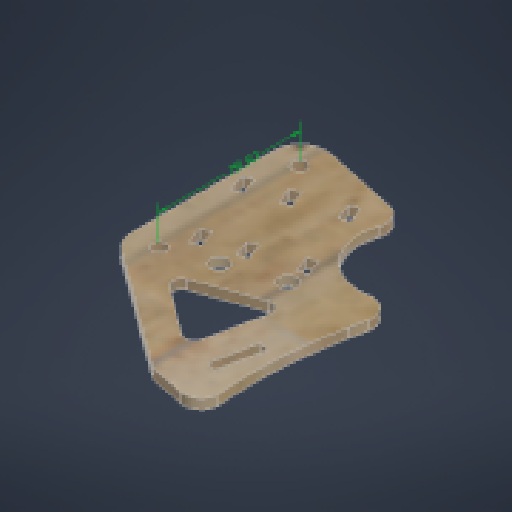
# Autodesk Inventor part: gear_plate_cover
Saved by Autodesk Inventor 2026.3 (Build 303398000, 398)
## iProperties
Created: 2024-04-01
Part Number: gear_plate_cover
Material: 木材 (カエデ材)
Document SubType Name: Modeling
Designer: hibik
Density: 0.67 g/cm^3
Appearance: ナチュラル カエデ材 - 光沢 濃い着色
Author: hibik
Autodesk Inventor part; units mm, degrees
ref_plane "YZ Plane" through (0, 0, 0) normal (1, 0, 0) x (0, 1, 0)
ref_plane "XZ Plane" through (0, 0, 0) normal (0, 1, 0) x (-1, 0, 0)
ref_plane "XY Plane" through (0, 0, 0) normal (0, 0, 1) x (1, 0, 0)
sketch "スケッチ1" plane through (0, 0, 0) normal (0, 1, 0) x (-1, 0, 0)
  line L0 (25, 0) -> (-25, 0)
  line L1 (-25, 0) -> (-25, -104.5)
  line L2 (-25, -104.5) -> (25, -104.5) construction
  line L3 (25, -104.5) -> (25, 0)
  circle A0 centre (0, 0) radius 25
  circle A1 centre (0, 0) radius 57 construction
  circle A2 centre (0, -79.5) radius 22.5 construction
  circle A3 centre (0, 0) radius 75 construction
  circle A4 centre (0, -79.5) radius 4
  circle A5 centre (0, 0) radius 4
  circle A6 centre (-77.7461, -62.8931) radius 25
  circle A7 centre (-77.7461, -62.8931) radius 10.75
  circle A8 centre (0, -79.5) radius 25
  line L4 (-5.2223, -103.9485) -> (-82.9684, -87.3415)
  line L5 (-72.5238, -38.4446) -> (5.2223, -55.0515)
  line L6 (-77.7461, -62.8931) -> (-82.9684, -87.3415)
  point P0 (25, -79.5)
  point P1 (-25, -48.5959)
  dimension "d0" = 114
  dimension "d1" = 45
  dimension "d2" = 150
  dimension "d4" = 8
  dimension "d5" = 50
  dimension "d25" = 79.5
  dimension "d41" = 8
  constraints: 14 end point, 9 centre point, 9 tangent, 8 coincident, 5 point on circle, 2 parallel, 2 perpendicular, 1 equal radius, 1 horizontal, 1 midpoint, 1 vertical alignment
  measures "d0" diameter of A1
  measures "d1" diameter of A2
  measures "d2" diameter of A3
  measures "d4" diameter of A5
  measures "d5" distance of L1.end L2.end
  measures "d25" distance from line of A2.centre L6
  measures "d41" diameter of A4
extrude "押し出し1" add sketch "スケッチ1" along normal blind 5.5 contours A0 L0 A5 | L0 A5 A0 | L3 A8 L5 L1 A0 | A8 | A8 L1 L5 | L4 L1 A8 | L1 L4 A6 L5 | A6
fillet "フィレット1" radius 5 1 edges at (25, 2.75, -48.5959)
sketch "スケッチ7" plane through (0, 5.5, 0) normal (0, 1, 0) x (1, 0, 0)
  circle A0 centre (0, 0) radius 4 projected
  circle A1 centre (0, 0) radius 15
  circle A2 centre (0, 79.5) radius 4 projected
  circle A3 centre (0, 79.5) radius 15
  line L0 (-15, 0) -> (-15, 79.5)
  line L1 (15, 79.5) -> (15, 0)
  arc A4 (-25, 0) -> (25, 0) centre (0, 0) ccw projected
  line L2 (25, 0) -> (25, 42.4151) projected
  arc A5 (31.0445, 47.3048) -> (25, 42.4151) centre (30, 42.4151) ccw projected
  line L3 (31.0445, 47.3048) -> (72.5238, 38.4446) projected
  arc A6 (72.5238, 38.4446) -> (82.9684, 87.3415) centre (77.7461, 62.8931) ccw projected
  line L4 (82.9684, 87.3415) -> (5.2223, 103.9485) projected
  arc A7 (5.2223, 103.9485) -> (-25, 79.5) centre (0, 79.5) ccw projected
  line L5 (-25, 79.5) -> (-25, 0) projected
  circle A8 centre (0, 0) radius 4 projected
  circle A9 centre (77.7461, 62.8931) radius 10.75 projected
  circle A10 centre (0, 79.5) radius 4 projected
  circle A11 centre (77.7461, 62.8931) radius 27.5
  line L6 (31.0445, 47.3048) -> (15, 50.732)
  line L7 (31.0445, 47.3048) -> (72.5238, 38.4446) projected
  line L8 (3.1334, 94.1691) -> (58.3391, 82.3769)
  point P0 (71.7647, 89.7347)
  dimension "d45" = 55
  dimension "d42" = 30
  constraints: 8 end point, 5 point on circle, 5 tangent, 3 coincident, 2 centre point, 1 collinear, 1 equal radius, 1 parallel, 1 point on line, 3 other
  measures "d42" diameter of A1
extrude "押し出し7" cut sketch "スケッチ7" against normal through all contours L1 L6 A5 L2 A4 L5 A7 L4 A11 L8 A3 L0 A1 | A11 L4 A6 L3 | L3 A6 L4 A11
sketch "スケッチ8" plane through (0, 5.5, 0) normal (0, 1, 0) x (1, 0, 0)
  circle A0 centre (84.2925, 23.2779) radius 1.6
  circle A1 centre (74.4966, 25.2879) radius 1.6
  arc A2 (18.2382, 101.1445) -> (16.4675, 97.727) centre (17.8362, 99.1853) ccw
  arc A3 (24.3587, 79.6988) -> (16.4675, 97.727) centre (-0.6405, 79.4974) ccw
  line L0 (24.3587, 79.6988) -> (24.5158, 60.1995)
  arc A4 (61.585, 20.7915) -> (24.5158, 60.1995) centre (0, 0) ccw
  line L1 (61.585, 20.7915) -> (92.6814, 14.4107)
  line L2 (92.6814, 14.4107) -> (101.7267, 58.4922)
  arc A5 (101.7267, 58.4922) -> (82.2621, 88.0071) centre (77.2369, 63.5174) ccw
  line L3 (82.2621, 88.0071) -> (18.2382, 101.1445)
  circle A6 centre (77.2369, 63.5174) radius 10.75
  line L4 (15, 50.732) -> (61.3201, 40.8378)
  arc A7 (58.3391, 82.3769) -> (61.3201, 40.8378) centre (77.7461, 62.8931) ccw
  line L5 (58.3391, 82.3769) -> (3.1334, 94.1691)
  arc A8 (3.1334, 94.1691) -> (-15, 79.5) centre (0, 79.5) ccw
  line L6 (-15, 79.5) -> (-15, 0)
  arc A9 (-15, 0) -> (15, 0) centre (0, 0) ccw
  line L7 (15, 0) -> (15, 50.732)
  circle A10 centre (0, 0) radius 4
  circle A11 centre (0, 79.5) radius 4
  circle A12 centre (77.7461, 62.8931) radius 27.5
  point P0 (99.0653, 45.5224)
  point P1 (48.1651, 43.6478)
  constraints: 18 centre point, 16 end point, 14 point on circle, 1 coincident
extrude "押し出し8" add sketch "スケッチ8" against normal up to surface (5.5 mm away) contours A0 | A1 | L2 L1 A4 L4 A12
sketch "スケッチ9" plane through (0, 5.5, 0) normal (0, 1, 0) x (1, 0, 0)
  circle A0 centre (77.1488, 63.6244) radius 4 projected
  line L0 (77.1488, 63.6244) -> (-2.7251, 34.5527)
  line L1 (10.9938, 12.9415) -> (5.8254, 11.0603)
  line L2 (5.8254, 11.0603) -> (-11.2756, 58.045)
  line L3 (-11.2756, 58.045) -> (-6.1073, 59.9261)
  line L4 (-6.1073, 59.9261) -> (10.9938, 12.9415)
  line L5 (-50.5492, 0) -> (128.2954, 0) projected
  line L6 (7.5735, 22.3384) -> (2.4052, 20.4573)
  line L7 (-7.8554, 48.6481) -> (-2.6871, 50.5292)
  point P0 (0, 0)
  dimension "d48" = 50
  dimension "d49" = 5.5
  dimension "d50" = 85
  dimension "d51" = 20
  dimension "d52" = 10
  dimension "d53" = 10
  constraints: 14 end point, 4 perpendicular, 4 point on line, 2 parallel, 1 midpoint
  measures "d48" distance between parallel lines of L3 L1
  measures "d49" distance between parallel lines of L2 L4
  measures "d50" distance from line of L0.start L2
  measures "d51" angle of L5 L0
  measures "d52" distance from line of L1.start L6
  measures "d53" distance from line of L3 L7.end
extrude "押し出し9" cut sketch "スケッチ9" against normal through all contours L7 L2 L3 L4 | L4 L1 L2 L6
sketch "スケッチ10" plane through (0, 5.5, 0) normal (0, 1, 0) x (1, 0, 0)
  line L0 (99.0653, 45.5224) -> (92.6814, 14.4107) projected
  line L1 (92.6814, 14.4107) -> (4.6453, -14.2626)
  arc A0 (-15, 0) -> (15, 0) centre (0, 0) ccw projected
  line L2 (2.4052, 20.4573) -> (7.5735, 22.3384) projected
  line L3 (7.5735, 22.3384) -> (10.9938, 12.9415) projected
  line L4 (10.9938, 12.9415) -> (5.8254, 11.0603) projected
  line L5 (5.8254, 11.0603) -> (2.4052, 20.4573) projected
  line L6 (-2.6871, 50.5292) -> (-7.8554, 48.6481) projected
  line L7 (-7.8554, 48.6481) -> (-11.2756, 58.045) projected
  line L8 (-11.2756, 58.045) -> (-6.1073, 59.9261) projected
  line L9 (-6.1073, 59.9261) -> (-2.6871, 50.5292) projected
  line L10 (15, 50.732) -> (48.1651, 43.6478) projected
  arc A1 (61.585, 20.7915) -> (48.1651, 43.6478) centre (0, 0) ccw projected
  line L11 (61.585, 20.7915) -> (92.6814, 14.4107) projected
  line L12 (92.6814, 14.4107) -> (99.0653, 45.5224) projected
  arc A2 (58.3391, 82.3769) -> (99.0653, 45.5224) centre (77.7461, 62.8931) ccw projected
  line L13 (58.3391, 82.3769) -> (3.1334, 94.1691) projected
  arc A3 (3.1334, 94.1691) -> (-15, 79.5) centre (0, 79.5) ccw projected
  line L14 (-15, 79.5) -> (-15, 0) projected
  arc A4 (-15, 0) -> (15, 0) centre (0, 0) ccw projected
  line L15 (15, 0) -> (15, 50.732) projected
  circle A5 centre (0, 0) radius 4 projected
  circle A6 centre (0, 79.5) radius 4 projected
  point P0 (92.6814, 14.4107)
  point P1 (15, 0)
  constraints: 2 end point, 1 point on circle, 1 tangent
extrude "押し出し10" add sketch "スケッチ10" against normal up to surface (5.5 mm away) contours L1 A0 L15 L10 A1 L11
sketch "スケッチ11" plane through (0, 5.5, 0) normal (0, 1, 0) x (1, 0, 0)
  line L0 (27.3071, 29.5208) -> (30.7273, 20.1239) projected
  line L1 (30.7273, 20.1239) -> (25.559, 18.2428) projected
  line L2 (22.1388, 27.6397) -> (25.559, 18.2428) projected
  line L3 (27.3071, 29.5208) -> (22.1388, 27.6397) projected
  line L4 (13.6263, 67.1085) -> (17.0465, 57.7116) projected
  line L5 (17.0465, 57.7116) -> (11.8782, 55.8305) projected
  line L6 (8.458, 65.2274) -> (11.8782, 55.8305) projected
  line L7 (13.6263, 67.1085) -> (8.458, 65.2274) projected
  line L8 (49.991, 27.1353) -> (46.5708, 36.5322) projected
  line L9 (46.5708, 36.5322) -> (51.7391, 38.4133) projected
  line L10 (55.1593, 29.0164) -> (51.7391, 38.4133) projected
  line L11 (49.991, 27.1353) -> (55.1593, 29.0164) projected
  line L12 (41.5219, 66.6199) -> (38.1017, 76.0168) projected
  line L13 (36.3102, 64.723) -> (32.89, 74.1199) projected
  line L14 (32.89, 74.1199) -> (38.0583, 76.001) projected
  line L15 (41.4785, 66.6041) -> (38.0583, 76.001) projected
  line L16 (36.3102, 64.723) -> (41.4785, 66.6041) projected
  point P0 (0, 0)
extrude "押し出し11" cut sketch "スケッチ11" against normal through all
fillet "フィレット2" radius 10 2 edges at (58.3391, 2.75, -82.3769) (99.0653, 2.75, -45.5224)
sketch "スケッチ12" plane through (0, 5.5, 0) normal (0, 1, 0) x (1, 0, 0)
  circle A0 centre (53.368, 19.3189) radius 5 projected
  circle A1 centre (25.1772, 9.0583) radius 5 projected
  point P0 (0, 0)
extrude "押し出し12" cut sketch "スケッチ12" against normal through all
sketch "スケッチ13" plane through (0, 5.5, 0) normal (0, 1, 0) x (1, 0, 0)
  line L0 (57.0478, -60.6098) -> (76.7295, -64.6199) projected
  arc A0 (76.7295, -64.6199) -> (88.6615, -55.9553) centre (78.726, -54.8212) ccw projected
  line L1 (88.6615, -55.9553) -> (101.9875, 60.7891) projected
  line L2 (4.6453, -14.2626) -> (92.6814, 14.4107) projected
  line L3 (92.6814, 14.4107) -> (94.6624, 24.0652) projected
  arc A1 (94.6624, 24.0652) -> (82.9678, 35.8934) centre (84.8665, 26.0753) ccw projected
  arc A2 (92.6814, 14.4107) -> (88.6615, -55.9553) centre (331.0724, -34.506) ccw
  arc A3 (-15, 0) -> (4.6453, -14.2626) centre (0, 0) ccw projected
  line L4 (57.0478, -60.6098) -> (-8.8911, -12.0809)
  constraints: 3 point on circle, 2 end point, 2 tangent, 1 centre point
extrude "押し出し13" add sketch "スケッチ13" against normal up to surface (5.5 mm away)
sketch "スケッチ14" plane through (0, 5.5, 0) normal (0, 1, 0) x (1, 0, 0)
  line L0 (70.4339, -42.9263) -> (75.8232, -44.0243)
  line L1 (75.8232, -44.0243) -> (80.8144, -19.5276)
  line L2 (80.8144, -19.5276) -> (75.4251, -18.4296)
  line L3 (75.4251, -18.4296) -> (70.4339, -42.9263)
  line L4 (57.0478, -60.6098) -> (76.7295, -64.6199) projected
  point P0 (0, 0)
  dimension "d65" = 5.5
  dimension "d66" = 25
  dimension "d67" = 5
  dimension "d68" = 20
  constraints: 8 end point, 3 parallel, 1 perpendicular
  measures "d65" distance between parallel lines of L1 L3
  measures "d66" distance between parallel lines of L0 L2
  measures "d67" distance from line of L4.end L1
  measures "d68" distance between parallel lines of L4 L0
extrude "押し出し14" cut sketch "スケッチ14" against normal through all
sketch "スケッチ15" plane through (0, 5.5, 0) normal (0, 1, 0) x (1, 0, 0)
  line L0 (14.6082, -10.7512) -> (55.5431, -40.8778)
  line L1 (14.6082, -10.7512) -> (65.4519, 7.7544)
  line L2 (65.4519, 7.7544) -> (55.5431, -40.8778)
  line L3 (-8.8911, -12.0809) -> (57.0478, -60.6098) projected
  line L4 (70.4339, -42.9263) -> (75.4251, -18.4296) projected
  circle A0 centre (53.368, 19.3189) radius 5 projected
  circle A1 centre (25.1772, 9.0583) radius 5 projected
  line L5 (25.1772, 9.0583) -> (53.368, 19.3189)
  point P0 (0, 0)
  dimension "d71" = 15
  dimension "d72" = 15
  dimension "d73" = 15
  constraints: 8 end point, 3 parallel
  measures "d71" distance between parallel lines of L3 L0
  measures "d72" distance between parallel lines of L5 L1
  measures "d73" distance between parallel lines of L4 L2
extrude "押し出し15" cut sketch "スケッチ15" against normal through all contours L1 L2 L0
fillet "フィレット3" radius 5 3 edges at (65.4519, 2.75, -7.7544) (14.6082, 2.75, 10.7512) (55.5431, 2.75, 40.8778)
equation "\"d73\" = d71"
